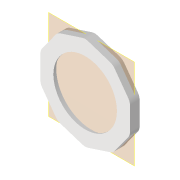
# Autodesk Inventor part: Anglerfish_Lightplate_rotator
Saved by Autodesk Inventor 2022 (Build 260153000, 153)
## iProperties
Created: 2022-10-04
Part Number: Anglerfish_Lightplate_rotator
Material: Generisch
Document SubType Name: Modeling
Designer: UC2
Density: 1 g/cm^3
Appearance: Vorgabe
Author: UC2
Autodesk Inventor part; units mm, degrees
ref_plane "YZ Plane" through (0, 0, 0) normal (1, 0, 0) x (0, 1, 0)
ref_plane "XZ Plane" through (0, 0, 0) normal (0, 1, 0) x (-1, 0, 0)
ref_plane "XY Plane" through (0, 0, 0) normal (0, 0, 1) x (1, 0, 0)
ref_plane "Arbeitsebene1" through (0, 0, 0) normal (0, 0, 1) x (1, 0, 0)
sketch "Skizze1" plane through (0, 0, 0) normal (0, 0, 1) x (1, 0, 0)
  arc A0 (-34.5, -10.235) -> (-33.9271, -11.9983) centre (-31.5, -10.235) ccw projected
  line L0 (-21.8951, -28.5589) -> (-33.9271, -11.9983) projected
  arc A1 (-21.8951, -28.5589) -> (-20.3951, -29.6487) centre (-19.4681, -26.7955) ccw projected
  line L1 (-0.9271, -35.9742) -> (-20.3951, -29.6487) projected
  arc A2 (-0.9271, -35.9742) -> (0.9271, -35.9742) centre (0, -33.1211) ccw projected
  line L2 (20.3951, -29.6487) -> (0.9271, -35.9742) projected
  arc A3 (20.3951, -29.6487) -> (21.8951, -28.5589) centre (19.4681, -26.7955) ccw projected
  line L3 (33.9271, -11.9983) -> (21.8951, -28.5589) projected
  arc A4 (33.9271, -11.9983) -> (34.5, -10.235) centre (31.5, -10.235) ccw projected
  line L4 (34.5, 10.235) -> (34.5, -10.235) projected
  arc A5 (34.5, 10.235) -> (33.9271, 11.9983) centre (31.5, 10.235) ccw projected
  line L5 (21.8951, 28.5589) -> (33.9271, 11.9983) projected
  arc A6 (21.8951, 28.5589) -> (20.3951, 29.6487) centre (19.4681, 26.7955) ccw projected
  line L6 (0.9271, 35.9742) -> (20.3951, 29.6487) projected
  arc A7 (0.9271, 35.9742) -> (-0.9271, 35.9742) centre (0, 33.1211) ccw projected
  line L7 (-20.3951, 29.6487) -> (-0.9271, 35.9742) projected
  arc A8 (-20.3951, 29.6487) -> (-21.8951, 28.5589) centre (-19.4681, 26.7955) ccw projected
  line L8 (-33.9271, 11.9983) -> (-21.8951, 28.5589) projected
  arc A9 (-33.9271, 11.9983) -> (-34.5, 10.235) centre (-31.5, 10.235) ccw projected
  line L9 (-34.5, -10.235) -> (-34.5, 10.235) projected
  arc A10 (2.4721, 40.7295) -> (-2.4721, 40.7295) centre (0, 33.1211) ccw
  line L10 (2.4721, 40.7295) -> (21.9402, 34.404)
  arc A11 (25.9402, 31.4978) -> (21.9402, 34.404) centre (19.4681, 26.7955) ccw
  line L11 (25.9402, 31.4978) -> (37.9721, 14.9373)
  arc A12 (39.5, 10.235) -> (37.9721, 14.9373) centre (31.5, 10.235) ccw
  line L12 (39.5, 10.235) -> (39.5, -10.235)
  arc A13 (37.9721, -14.9373) -> (39.5, -10.235) centre (31.5, -10.235) ccw
  line L13 (37.9721, -14.9373) -> (25.9402, -31.4978)
  arc A14 (21.9402, -34.404) -> (25.9402, -31.4978) centre (19.4681, -26.7955) ccw
  line L14 (21.9402, -34.404) -> (2.4721, -40.7295)
  arc A15 (-2.4721, -40.7295) -> (2.4721, -40.7295) centre (0, -33.1211) ccw
  line L15 (-2.4721, -40.7295) -> (-21.9402, -34.404)
  arc A16 (-25.9402, -31.4978) -> (-21.9402, -34.404) centre (-19.4681, -26.7955) ccw
  line L16 (-25.9402, -31.4978) -> (-37.9721, -14.9373)
  arc A17 (-39.5, -10.235) -> (-37.9721, -14.9373) centre (-31.5, -10.235) ccw
  line L17 (-39.5, -10.235) -> (-39.5, 10.235)
  arc A18 (-37.9721, 14.9373) -> (-39.5, 10.235) centre (-31.5, 10.235) ccw
  line L18 (-37.9721, 14.9373) -> (-25.9402, 31.4978)
  arc A19 (-21.9402, 34.404) -> (-25.9402, 31.4978) centre (-19.4681, 26.7955) ccw
  line L19 (-21.9402, 34.404) -> (-2.4721, 40.7295)
  circle A20 centre (0, 0) radius 27.2618 projected
  circle A21 centre (0, 0) radius 30 projected
  circle A22 centre (0, 0) radius 31
  point P0 (0, 0)
  dimension "d0" = 5
  dimension "d1" = 1
  constraints: 20 end point, 20 point on circle, 11 centre point, 19 other
  measures "d0" distance between parallel lines of L7 L19
  measures "d1" radial gap between concentric circles of A21 A22
extrude "Extrusion1" add sketch "Skizze1" along normal blind 4.5 contours L9 A9 L8 A8 L7 A7 L6 A6 L5 A5 L4 A4 L3 A3 L2 A2 L1 A1 L0 A0 | L10 A11 L11 A12 L12 A13 L13 A14 L14 A15 L15 A16 L16 A17 L17 A18 L18 A19 L19 A10
sketch "Skizze2" plane through (0, 0, 4.5) normal (0, 0, 1) x (1, 0, 0)
  line L0 (21.9402, 34.404) -> (2.4721, 40.7295) projected
  arc A0 (2.4721, 40.7295) -> (-2.4721, 40.7295) centre (0, 33.1211) ccw projected
  line L1 (-2.4721, 40.7295) -> (-21.9402, 34.404) projected
  arc A1 (-21.9402, 34.404) -> (-25.9402, 31.4978) centre (-19.4681, 26.7955) ccw projected
  line L2 (-25.9402, 31.4978) -> (-37.9721, 14.9373) projected
  arc A2 (-37.9721, 14.9373) -> (-39.5, 10.235) centre (-31.5, 10.235) ccw projected
  line L3 (-39.5, 10.235) -> (-39.5, -10.235) projected
  arc A3 (-39.5, -10.235) -> (-37.9721, -14.9373) centre (-31.5, -10.235) ccw projected
  line L4 (-37.9721, -14.9373) -> (-25.9402, -31.4978) projected
  arc A4 (-25.9402, -31.4978) -> (-21.9402, -34.404) centre (-19.4681, -26.7955) ccw projected
  line L5 (-21.9402, -34.404) -> (-2.4721, -40.7295) projected
  arc A5 (-2.4721, -40.7295) -> (2.4721, -40.7295) centre (0, -33.1211) ccw projected
  line L6 (2.4721, -40.7295) -> (21.9402, -34.404) projected
  arc A6 (21.9402, -34.404) -> (25.9402, -31.4978) centre (19.4681, -26.7955) ccw projected
  line L7 (25.9402, -31.4978) -> (37.9721, -14.9373) projected
  arc A7 (37.9721, -14.9373) -> (39.5, -10.235) centre (31.5, -10.235) ccw projected
  line L8 (39.5, -10.235) -> (39.5, 10.235) projected
  arc A8 (39.5, 10.235) -> (37.9721, 14.9373) centre (31.5, 10.235) ccw projected
  line L9 (37.9721, 14.9373) -> (25.9402, 31.4978) projected
  arc A9 (25.9402, 31.4978) -> (21.9402, 34.404) centre (19.4681, 26.7955) ccw projected
  circle A10 centre (0, 0) radius 31 projected
  circle A11 centre (0, 0) radius 28
  point P0 (0, 0)
  dimension "d4" = 3
  constraints: 1 centre point
  measures "d4" radial gap between concentric circles of A10 A11
extrude "Extrusion2" add sketch "Skizze2" along normal blind 1 contours A9 L9 A8 L8 A7 L7 A6 L6 A5 L5 A4 L4 A3 L3 A2 L2 A1 L1 A0 L0 | A10
sketch "Skizze3" plane through (0, 0, 0) normal (0, 0, -1) x (-1, 0, 0)
  line L0 (21.8951, -28.5589) -> (33.9271, -11.9983) projected
  line L1 (35.7634, -13.3325) -> (23.7315, -29.893) projected
  line L2 (-21.9402, 34.404) -> (-2.4721, 40.7295) projected
  arc A0 (-21.9402, 34.404) -> (-25.9402, 31.4978) centre (-19.4681, 26.7955) ccw projected
  line L3 (-37.9721, 14.9373) -> (-25.9402, 31.4978) projected
  arc A1 (-37.9721, 14.9373) -> (-39.5, 10.235) centre (-31.5, 10.235) ccw projected
  line L4 (-39.5, -10.235) -> (-39.5, 10.235) projected
  arc A2 (-39.5, -10.235) -> (-37.9721, -14.9373) centre (-31.5, -10.235) ccw projected
  line L5 (-25.9402, -31.4978) -> (-37.9721, -14.9373) projected
  arc A3 (-25.9402, -31.4978) -> (-21.9402, -34.404) centre (-19.4681, -26.7955) ccw projected
  line L6 (-2.4721, -40.7295) -> (-21.9402, -34.404) projected
  arc A4 (-2.4721, -40.7295) -> (2.4721, -40.7295) centre (0, -33.1211) ccw projected
  line L7 (21.9402, -34.404) -> (2.4721, -40.7295) projected
  arc A5 (21.9402, -34.404) -> (25.9402, -31.4978) centre (19.4681, -26.7955) ccw projected
  line L8 (37.9721, -14.9373) -> (25.9402, -31.4978) projected
  arc A6 (37.9721, -14.9373) -> (39.5, -10.235) centre (31.5, -10.235) ccw projected
  line L9 (39.5, 10.235) -> (39.5, -10.235) projected
  arc A7 (39.5, 10.235) -> (37.9721, 14.9373) centre (31.5, 10.235) ccw projected
  line L10 (25.9402, 31.4978) -> (37.9721, 14.9373) projected
  arc A8 (25.9402, 31.4978) -> (21.9402, 34.404) centre (19.4681, 26.7955) ccw projected
  line L11 (2.4721, 40.7295) -> (21.9402, 34.404) projected
  arc A9 (2.4721, 40.7295) -> (-2.4721, 40.7295) centre (0, 33.1211) ccw projected
  circle A10 centre (0, 0) radius 31 projected
  arc A11 (21.2295, -32.2165) -> (24.0795, -30.1459) centre (19.4681, -26.7955) ccw
  line L12 (21.2295, -32.2165) -> (1.7614, -38.5421)
  arc A12 (-1.7614, -38.5421) -> (1.7614, -38.5421) centre (0, -33.1211) ccw
  line L13 (-1.7614, -38.5421) -> (-21.2295, -32.2165)
  arc A13 (-24.0795, -30.1459) -> (-21.2295, -32.2165) centre (-19.4681, -26.7955) ccw
  line L14 (-24.0795, -30.1459) -> (-36.1114, -13.5853)
  arc A14 (-37.2, -10.235) -> (-36.1114, -13.5853) centre (-31.5, -10.235) ccw
  line L15 (-37.2, -10.235) -> (-37.2, 10.235)
  arc A15 (-36.1114, 13.5853) -> (-37.2, 10.235) centre (-31.5, 10.235) ccw
  line L16 (-36.1114, 13.5853) -> (-24.0795, 30.1459)
  arc A16 (-21.2295, 32.2165) -> (-24.0795, 30.1459) centre (-19.4681, 26.7955) ccw
  line L17 (-21.2295, 32.2165) -> (-1.7614, 38.5421)
  arc A17 (1.7614, 38.5421) -> (-1.7614, 38.5421) centre (0, 33.1211) ccw
  line L18 (1.7614, 38.5421) -> (21.2295, 32.2165)
  arc A18 (24.0795, 30.1459) -> (21.2295, 32.2165) centre (19.4681, 26.7955) ccw
  line L19 (24.0795, 30.1459) -> (36.1114, 13.5853)
  arc A19 (37.2, 10.235) -> (36.1114, 13.5853) centre (31.5, 10.235) ccw
  line L20 (37.2, 10.235) -> (37.2, -10.235)
  arc A20 (36.1114, -13.5853) -> (37.2, -10.235) centre (31.5, -10.235) ccw
  line L21 (36.1114, -13.5853) -> (24.0795, -30.1459)
  point P0 (0, 0)
  dimension "d7" = 2.3
  constraints: 20 end point, 20 point on circle, 10 centre point, 19 other
  measures "d7" distance between parallel lines of L8 L21
extrude "Extrusion3" add sketch "Skizze3" along normal blind 3 contours L2 A9 L11 A8 L10 A7 L9 A6 L8 A5 L7 A4 L6 A3 L5 A2 L4 A1 L3 A0
